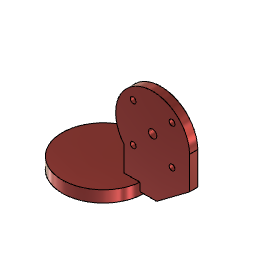
tampa-base-conectora (Autodesk Fusion 360 design; units mm, degrees)
Autodesk Fusion 360 part; units mm, degrees
sketch "Sketch1" plane through (0, 0, 0) normal (0, 0, 1) x (1, 0, 0)
  circle A0 centre (0, 0) radius 50
  circle A1 centre (0, 0) radius 3.25
  line L0 (1.7058, 2.7664) -> (-1.7058, 2.7664)
  dimension "d1" = 100
  dimension "d2" = 6.5
  constraint coincident A0.centre A1.centre
  constraint coincident A1 L0.start
  constraint coincident A1 L0.end
  constraint horizontal L0
  measures "d1" diameter of A0
  measures "d2" diameter of A1
extrude "Extrude1" add sketch "Sketch1" along normal blind 10 contours A0 | A1 L0 | A1 L0
extrude "Extrude2" cut sketch "Sketch1" along normal blind 7 contours A1 L0 picked at (0.999, 0.1306)
sketch "Sketch2" plane through (0, 0, 0) normal (0, 1, 0) x (1, 0, 0)
  line L0 (0, 20) -> (0, -60)
  line L1 (30, 20) -> (30, -40.4129)
  line L2 (110, 20) -> (110, -69.665)
  line L3 (-75, 0) -> (110, 0)
  line L4 (-75, -60) -> (115, -60)
  line L5 (90, -50) -> (130, -50)
  circle A0 centre (65.0107, -68.6839) radius 45
  circle A1 centre (65.0107, -68.6839) radius 5
  line L6 (88.6327, -92.3059) -> (41.3887, -92.3059)
  line L7 (41.3887, -92.3059) -> (41.3887, -45.0619)
  line L8 (41.3887, -45.0619) -> (88.6327, -45.0619)
  line L9 (88.6327, -45.0619) -> (88.6327, -92.3059)
  line L10 (88.6327, -92.3059) -> (41.3887, -45.0619) construction
  line L11 (41.3887, -92.3059) -> (88.6327, -45.0619) construction
  circle A2 centre (41.3887, -45.0619) radius 3.5
  circle A3 centre (88.6327, -45.0619) radius 3.5
  circle A4 centre (41.3887, -92.3059) radius 3.5
  circle A5 centre (88.6327, -92.3059) radius 3.5
  line L12 (110, -30) -> (70, 0)
  point P0 (65.0107, -68.6839)
  dimension "d7" = 30
  dimension "d8" = 80
  dimension "d9" = 60
  dimension "d10" = 50
  dimension "d11" = 90
  dimension "d12" = 10
  dimension "d13" = 47.244
  dimension "d14" = 47.244
  dimension "d15" = 7
  dimension "d16" = 7
  dimension "d17" = 7
  dimension "d18" = 7
  constraint vertical L0
  constraint vertical L1
  constraint vertical L2
  constraint coincident L2 L3.end
  constraint perpendicular L2 L3
  constraint perpendicular L2 L4
  constraint perpendicular L2 L5
  constraint coincident L2.end A0
  constraint concentric A0 A1
  constraint coincident L1.end A0
  constraint horizontal L6
  constraint perpendicular L6 L7
  constraint parallel L6 L8
  constraint parallel L7 L9
  constraint coincident L10 P0
  constraint coincident L11 P0
  constraint coincident P0 A0.centre
  constraint coincident L7.end L8.start
  constraint coincident L8.end L9.start
  constraint coincident L6.end L7.start
  constraint coincident L6.start L9.end
  constraint coincident L2 L12.start
  constraint coincident L3 L12.end
  measures "d7" distance of L0 L1
  measures "d8" distance of L1 L2
  measures "d9" distance of L3 L4
  measures "d10" distance of L3 L5
  measures "d11" diameter of A0
  measures "d12" diameter of A1
  measures "d13" distance of L7.end L8.end
  measures "d14" distance of L6 L8
  measures "d15" diameter of A2
  measures "d16" diameter of A3
  measures "d17" diameter of A4
  measures "d18" diameter of A5
extrude "Extrude3" add sketch "Sketch2" along normal mid plane 10 contours L1 L2 L3 L5 A0 L12 | L4 A0 L7 L8 L9 A2 A3 | L2 L4 A0 L6 L7 L9 A4 A5 | L4 L7 L8 L9 A2 A3 | L4 L6 L7 L9 A4 A5 | L2 L4 L5 A0 | L2 L4 A0
extrude "Extrude4" add sketch "Sketch1" against normal blind 4
component "6627T54_Stepper Motor (2)" placed x (1, 0, 0) y (0, 0, -1) z (0, 1, 0) at (-34.4133, -232.4903, 46.7909)
